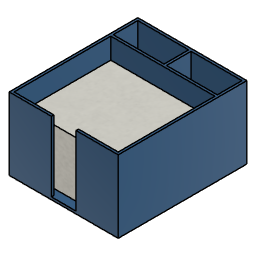
Paperholder-V1 (Autodesk Fusion 360 design; units mm, degrees)
Autodesk Fusion 360 part; units mm, degrees
sketch "Skizze1" plane through (0, 0, 0) normal (0, 0, 1) x (1, 0, 0)
  line L0 (-45, 50) -> (44, 50)
  line L1 (44, 50) -> (44, -55)
  line L2 (44, -55) -> (-45, -55)
  line L3 (-45, -55) -> (-45, 50)
  line L4 (-43, 48) -> (42, 48)
  line L5 (42, 48) -> (42, -53)
  line L6 (42, -53) -> (-43, -53)
  line L7 (-43, -53) -> (-43, 48)
  line L8 (-10.5, -53) -> (9.5, -53)
  line L9 (9.5, -53) -> (9.5, -55)
  line L10 (9.5, -55) -> (-10.5, -55)
  line L11 (-10.5, -55) -> (-10.5, -53)
  line L12 (-43, 27.9185) -> (42, 27.9185)
  line L13 (42, 27.9185) -> (42, 25.9185)
  line L14 (42, 25.9185) -> (-43, 25.9185)
  line L15 (-43, 25.9185) -> (-43, 27.9185)
  line L16 (-1.5, 48) -> (0.5, 48)
  line L17 (0.5, 48) -> (0.5, 27.9185)
  line L18 (0.5, 27.9185) -> (-1.5, 27.9185)
  line L19 (-1.5, 27.9185) -> (-1.5, 48)
  dimension "d1" = 89
  dimension "d2" = 105
  dimension "d3" = 2
  dimension "d4" = 2
  dimension "d5" = 2
  dimension "d6" = 2
  dimension "d7" = 20
  dimension "d8" = 34.5
  dimension "d9" = 34.5
  dimension "d10" = 2
  dimension "d11" = 2
  dimension "d12" = 41.5
  dimension "d13" = 85
  dimension "d14" = 41.5
  constraint horizontal L0
  constraint vertical L1
  constraint horizontal L2
  constraint vertical L3
  constraint horizontal L4
  constraint vertical L5
  constraint horizontal L6
  constraint vertical L7
  constraint horizontal L8
  constraint vertical L9
  constraint horizontal L10
  constraint vertical L11
  constraint coincident L2 L9.end
  constraint coincident L6 L8.start
  constraint horizontal L12
  constraint vertical L13
  constraint horizontal L14
  constraint vertical L15
  constraint coincident L5 L13.end
  constraint coincident L7 L12.start
  constraint horizontal L16
  constraint vertical L17
  constraint horizontal L18
  constraint vertical L19
  constraint coincident L12 L17.end
  constraint coincident L4 L16.start
  measures "d1" distance of L0.start L0.end
  measures "d2" distance of L0.start L2.end
  measures "d3" distance of L1 L5
  measures "d4" distance of L3 L7
  measures "d5" distance of L0 L4
  measures "d6" distance of L2 L6
  measures "d7" distance of L8.start L8.end
  measures "d8" distance of L3 L11
  measures "d9" distance of L1 L9
  measures "d10" distance of L16.start L16.end
  measures "d11" distance of L12 L14
  measures "d12" distance of L5 L17
  measures "d13" distance of L4.start L4.end
  measures "d14" distance of L7 L19
extrude "Extrusion1" add sketch "Skizze1" along normal blind 2 contours L5 L6 L7 L8 L14 | L4 L7 L12 L19 | L4 L5 L12 L17 makes body 1 at (13.6667, -26.6938, 0) makes body 2 at (28.1667, 34.6123, 0) makes body 3 at (-29.1667, 41.3062, 0)
extrude "Extrusion2" add sketch "Skizze1" along normal blind 59 contours L0 L1 L2 L3 L4 L5 L6 L7 L9 L11 L13 L15 L16 | L5 L7 L12 L13 L14 L15 L18 | L4 L12 L16 L17 L18 L19 bodies 1 2 3
extrude "Extrusion3" add 1 faces at (2.8333, -53, 0.6667) along direction (0, -1, 0) blind 2 on bodies 1 bodies 1
sketch "Skizze2" plane through (0, 0, 2) normal (0, 0, 1) x (-1, 0, 0)
  line L0 (-42, 53) -> (-42, -25.9185)
  line L1 (-42, -25.9185) -> (43, -25.9185)
  line L2 (43, -25.9185) -> (43, 53)
  line L3 (43, 53) -> (10.5, 53)
  line L4 (10.5, 53) -> (10.5, 55)
  line L5 (10.5, 55) -> (-9.5, 55)
  line L6 (-9.5, 55) -> (-9.5, 53)
  line L7 (-9.5, 53) -> (-42, 53)
  line L8 (38, -20.9185) -> (-37, -20.9185)
  line L9 (-37, -20.9185) -> (-37, 48)
  line L10 (-37, 48) -> (38, 48)
  line L11 (38, 48) -> (38, -20.9185)
  dimension "d21" = 5
  dimension "d22" = 5
  dimension "d23" = 5
  dimension "d24" = 5
  constraint horizontal L8
  constraint vertical L9
  constraint horizontal L10
  constraint vertical L11
  measures "d21" distance of L0 L9
  measures "d22" distance of L2 L11
  measures "d23" distance of L3 L10
  measures "d24" distance of L1 L8
extrude "Extrusion4" add sketch "Skizze2" along normal blind 45 separate body contours L8 L9 L10 L11 makes body 4
named bodies: "main", "sticky-notes"
